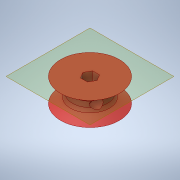
# Autodesk Inventor part: RoundShaftSpoolForArmV01
Saved by Autodesk Inventor 2022.2 (Build 262287010, 287A)
## iProperties
Created: 2019-02-24
Part Number: RoundShaftSpoolForArmV01
Material: PC/ABS Plastic
Document SubType Name: Modeling
Designer: steele
Density: 0.357273 g/cm^3
Appearance: Smooth - Red
holeForString: 0.200 in
stringDiameter: 0.120 in
clearanceForString: 0.080 in
clearanceForHexShaft: 0.020 in
spoolInteriorDiameter: 1.500 in
spoolInteriroRadius: 0.750 in
spoolExteriorDiameter: 2.500 in
spoolExteriorRadius: 1.250 in
hexHoleChamfer: 0.063 in
stringHoleCenterFromHexShaft: 0.360 in
textCircleDiameter: 1.875 in
textHeight: 0.180 in
textDepth: 0.050 in
Author: steele
Autodesk Inventor part; units mm, degrees
ref_plane "XZ Plane" through (0, 0, 0) normal (0, 1, 0) x (-1, 0, 0)
ref_plane "XY Plane" through (0, 0, 0) normal (0, 0, 1) x (1, 0, 0)
sketch "Sketch15" plane through (0, 0, 0) normal (0, 0, 1) x (1, 0, 0)
  line L0 (31.75, 0) -> (31.75, 50.8) construction
  line L1 (12.065, 0) -> (31.75, 0)
  line L2 (19.05, 0) -> (19.05, 50.8) construction
  line L3 (0, 50.8) -> (0, 0)
  line L4 (19.05, 12.7) -> (31.75, 12.7) construction
  line L5 (31.75, 0) -> (19.05, 7.3323)
  line L6 (31.75, 25.4) -> (19.05, 18.0677)
  line L7 (19.05, 18.0677) -> (31.75, 18.0677) construction
  line L8 (19.05, 18.0677) -> (19.05, 7.3323)
  line L9 (31.75, 25.4) -> (19.05, 32.7323)
  line L10 (19.05, 32.7323) -> (19.05, 43.4677)
  line L11 (19.05, 43.4677) -> (31.75, 50.8)
  line L12 (31.75, 25.4) -> (19.05, 25.4) construction
  line L13 (19.05, 43.4677) -> (31.75, 43.4677) construction
  line L14 (12.065, 0) -> (0, 0)
  line L15 (31.75, 50.8) -> (0, 50.8)
  dimension "d86" = 50.8
  dimension "d89" = 25.4
  dimension "centerLineForSpool" = 12.7
  dimension "d93" = 30
  dimension "d94" = 30
  dimension "d95" = 30
  dimension "d96" = 30
  dimension "d156" = 31.75
  dimension "d158" = 31.75
  constraints: 32 end point, 9 point on line, 3 horizontal, 2 midpoint, 2 perpendicular, 1 collinear, 1 vertical
  measures "d86" distance of L0.start L0.end
  measures "d89" distance from line of L6.start L1
  measures "centerLineForSpool" distance from line of L4.start L1
  measures "d93" angle of L5 L1
  measures "d94" angle of L6 L7
  measures "d95" angle of L9 L12
  measures "d96" angle of L11 L13
  measures "d156" distance from line of L0.end L3
  measures "d158" distance from line of L0.start L3
revolve "Revolution2" add sketch "Sketch15" angle 360 about axis through (0, 50.8, 0) along (0, -1, 0)
sketch "Sketch16" plane through (0, 0, 0) normal (0, -1, 0) x (1, 0, 0)
  line L0 (-7.6256, 0) -> (-3.8128, 6.604)
  line L1 (-3.8128, 6.604) -> (3.8128, 6.604)
  line L2 (3.8128, 6.604) -> (7.6256, 0)
  line L3 (7.6256, 0) -> (3.8128, -6.604)
  line L4 (3.8128, -6.604) -> (-3.8128, -6.604)
  line L5 (-3.8128, -6.604) -> (-7.6256, 0)
  point P0 (0, 0)
  point P1 (0, 0)
  dimension "d103" = 13.208
  constraints: 12 end point, 1 coincident, 1 horizontal, 13 other
  measures "d103" distance between parallel lines of L1 L4
extrude "Extrusion11" cut sketch "Sketch16" against normal through all
sketch "Sketch17" plane through (0, 0, 0) normal (1, 0, 0) x (0, 1, 0)
  circle A0 centre (38.1, 9.144) radius 2.54
  circle A1 centre (12.7, 9.144) radius 2.54
  line L0 (0, 31.75) -> (0, -31.75) projected
  line L1 (50.8, 31.75) -> (50.8, -31.75) projected
  line L2 (0, 6.604) -> (50.8, 6.604) projected
  point P0 (0, 0)
  point P1 (50.8, -31.75)
  point P2 (69.85, 6.858)
  point P3 (72.39, 6.858)
  point P4 (50.8, 6.604)
  dimension "d110" = 12.7
  dimension "d111" = 12.7
  dimension "d112" = 5.08
  constraints: 2 centre point, 1 equal radius, 4 other
  measures "d110" distance from line of A1.centre L0
  measures "d112" diameter of A0
extrude "Extrusion13" cut sketch "Sketch17" along normal through all both and the other way through all
ref_plane "Work Plane4" through (-19.05, 0, 0) normal (1, 0, 0) x (0, 1, 0)
sketch "Sketch22" plane through (-19.05, 0, 0) normal (1, 0, 0) x (0, 1, 0)
  spline S0 degree 8 poles (40.64, 9.144) (40.64, 9.42) (40.6057, 9.6896) (40.54, 9.9488) (40.4456, 10.1945) (40.3253, 10.4241) (40.1822, 10.6353) (40.019, 10.8263) (39.6643, 11.1594) (39.4723, 11.3044) (39.2651, 11.4282) (39.0456, 11.5293) (38.8165, 11.6061) (38.5806, 11.6579) (38.3408, 11.684) (37.8188, 11.684) (37.5395, 11.6484) (37.2666, 11.5781) (37.0042, 11.4743) (36.7566, 11.3384) (36.5278, 11.1726) (36.322, 10.9796) (35.9648, 10.5477) (35.8095, 10.305) (35.6834, 10.0377) (35.5915, 9.75) (35.5382, 9.4472) (35.5271, 9.1354) (35.5605, 8.8213) (35.7533, 8.0702) (35.9537, 7.6667) (36.2256, 7.316) (36.5542, 7.0287) (36.9234, 6.8124) (37.3159, 6.6712) (37.7136, 6.604) (38.3775, 6.604) (38.6564, 6.6386) (38.9325, 6.7085) (39.2015, 6.8141) (39.4588, 6.9552) (39.6993, 7.1318) (39.9175, 7.3429) (40.2331, 7.7498) (40.3461, 7.9265) (40.4431, 8.1154) (40.522, 8.3139) (40.5815, 8.5192) (40.6208, 8.7281) (40.64, 8.9374) (40.64, 9.144) knots 0 0 0 0 0 0 0 0 0 0.12897 0.12897 0.12897 0.12897 0.12897 0.12897 0.12897 0.253758 0.253758 0.253758 0.253758 0.253758 0.253758 0.253758 0.399502 0.399502 0.399502 0.399502 0.399502 0.399502 0.399502 0.544455 0.544455 0.544455 0.544455 0.544455 0.544455 0.544455 0.751871 0.751871 0.751871 0.751871 0.751871 0.751871 0.751871 0.90085 0.90085 0.90085 0.90085 0.90085 0.90085 0.90085 1 1 1 1 1 1 1 1 1 projected
  circle A0 centre (38.1, 9.144) radius 4.7625
  circle A1 centre (38.1, 9.144) radius 2.54 construction
  line L0 (38.1, 6.604) -> (12.7, 6.604) construction
  line L1 (50.8, 31.75) -> (50.8, -31.75) construction
  point P0 (0, 0)
  point P1 (69.85, 6.858)
  point P2 (50.8, -31.75)
  point P3 (72.39, 6.858)
  point P4 (12.7, 6.604)
  dimension "d121" = 12.7
  dimension "d122" = 5.08
  dimension "d125" = 9.525
  constraints: 2 centre point, 1 concentric, 1 vertical alignment, 3 other
  measures "d122" diameter of A1
  measures "d125" diameter of A0
extrude "Extrusion16" cut sketch "Sketch22" along normal blind 11.1125
ref_plane "Work Plane5" through (19.05, 0, 0) normal (1, 0, 0) x (0, 1, 0)
sketch "Sketch23" plane through (19.05, 0, 0) normal (1, 0, 0) x (0, 1, 0)
  line L0 (12.7, 6.604) -> (38.1, 6.604) projected
  circle A0 centre (12.7, 9.144) radius 2.54 construction
  line L1 (0, 31.75) -> (0, -31.75) projected
  circle A1 centre (12.7, 9.144) radius 4.7625
  point P0 (0, 0)
  dimension "d127" = 5.08
  dimension "d128" = 12.7
  dimension "d129" = 9.525
  constraints: 2 centre point, 1 coincident, 1 tangent
  measures "d127" diameter of A0
  measures "d128" distance from line of A0.centre L1
  measures "d129" diameter of A1
extrude "Extrusion17" cut sketch "Sketch23" against normal blind 11.1125
chamfer "Chamfer12" distance 2.3813 angle 45 4 edges at (-19.05, 43.4677, 0) (-19.05, 32.7323, 0) (-19.05, 18.0677, 0) (-19.05, 7.3323, 0)
ref_plane "Work Plane6" through (0, 25.4, 0) normal (0, -1, 0) x (1, 0, 0)
sketch "Sketch26" plane through (0, 0, 0) normal (0, -1, 0) x (1, 0, 0)
  circle A0 centre (0, 0) radius 23.8125 construction
  line L0 (-23.5941, 3.5966) -> (-23.6743, 2.6429)
  line L1 (-23.6743, 2.6429) -> (-25.3572, 2.7844)
  line L2 (-25.3572, 2.7844) -> (-25.4662, 1.4891)
  line L3 (-25.4662, 1.4891) -> (-23.7832, 1.3476)
  line L4 (-23.7832, 1.3476) -> (-23.8634, 0.3938)
  line L5 (-23.8634, 0.3938) -> (-27.66, 0.713)
  line L6 (-27.66, 0.713) -> (-27.5798, 1.6668)
  line L7 (-27.5798, 1.6668) -> (-26.1892, 1.5499)
  line L8 (-26.1892, 1.5499) -> (-26.0803, 2.8452)
  line L9 (-26.0803, 2.8452) -> (-27.4709, 2.9621)
  line L10 (-27.4709, 2.9621) -> (-27.3907, 3.9159)
  line L11 (-27.3907, 3.9159) -> (-23.5941, 3.5966)
  spline S0 degree 2 poles (-23.0339, 5.7334) (-23.2221, 4.9404) (-24.1795, 4.2759) (-24.8794, 4.442) knots 0 0 0 1 2 2 2
  spline S1 degree 2 poles (-24.8794, 4.442) (-25.5644, 4.6046) (-26.1947, 5.5856) (-26.0264, 6.2946) knots 0 0 0 1 2 2 2
  spline S2 degree 2 poles (-26.0264, 6.2946) (-25.8745, 6.9344) (-25.0266, 7.4186) (-24.3837, 7.266) knots 0 0 0 1 2 2 2
  line L12 (-24.3837, 7.266) -> (-24.0683, 7.1912)
  line L13 (-24.0683, 7.1912) -> (-24.5225, 5.2776)
  spline S3 degree 2 poles (-24.5225, 5.2776) (-24.3244, 5.2432) (-24.0325, 5.3231) (-23.9273, 5.4187) knots 0 0 0 1 2 2 2
  spline S4 degree 2 poles (-23.9273, 5.4187) (-23.8228, 5.5113) (-23.6854, 5.7961) (-23.6433, 5.9733) knots 0 0 0 1 2 2 2
  spline S5 degree 2 poles (-23.6433, 5.9733) (-23.6077, 6.1235) (-23.6039, 6.4336) (-23.6318, 6.5703) knots 0 0 0 1 2 2 2
  spline S6 degree 2 poles (-23.6318, 6.5703) (-23.6512, 6.6891) (-23.7195, 6.8958) (-23.748, 6.9628) knots 0 0 0 1 2 2 2
  line L14 (-23.748, 6.9628) -> (-23.7259, 7.056)
  line L15 (-23.7259, 7.056) -> (-23.005, 6.8848)
  spline S7 degree 2 poles (-23.005, 6.8848) (-22.9886, 6.7667) (-22.9578, 6.5754) (-22.9589, 6.4106) knots 0 0 0 1 2 2 2
  spline S8 degree 2 poles (-22.9589, 6.4106) (-22.9533, 6.2601) (-22.9825, 5.9497) (-23.0339, 5.7334) knots 0 0 0 1 2 2 2
  spline S9 degree 2 poles (-24.7979, 6.4568) (-25.0757, 6.5164) (-25.4249, 6.3422) (-25.484, 6.0928) knots 0 0 0 1 2 2 2
  spline S10 degree 2 poles (-25.484, 6.0928) (-25.5446, 5.8375) (-25.3067, 5.4764) (-25.0489, 5.3993) knots 0 0 0 1 2 2 2
  line L16 (-25.0489, 5.3993) -> (-24.7979, 6.4568)
  line L17 (-21.6776, 9.9814) -> (-22.0524, 9.0008)
  line L18 (-22.0524, 9.0008) -> (-23.0175, 8.7846)
  line L19 (-23.0175, 8.7846) -> (-22.4481, 7.9654)
  line L20 (-22.4481, 7.9654) -> (-22.8152, 7.005)
  line L21 (-22.8152, 7.005) -> (-23.781, 8.508)
  line L22 (-23.781, 8.508) -> (-25.4936, 8.0486)
  line L23 (-25.4936, 8.0486) -> (-25.1188, 9.0292)
  line L24 (-25.1188, 9.0292) -> (-24.1714, 9.2422)
  line L25 (-24.1714, 9.2422) -> (-24.7341, 10.0357)
  line L26 (-24.7341, 10.0357) -> (-24.367, 10.9961)
  line L27 (-24.367, 10.9961) -> (-23.4176, 9.5193)
  line L28 (-23.4176, 9.5193) -> (-21.6776, 9.9814)
  line L29 (-22.6697, 14.9203) -> (-22.7047, 14.8621)
  spline S11 degree 2 poles (-22.7047, 14.8621) (-22.745, 14.825) (-22.9002, 14.6625) (-22.9495, 14.5805) knots 0 0 0 1 2 2 2
  spline S12 degree 2 poles (-22.9495, 14.5805) (-23.0894, 14.3476) (-23.0218, 14.0764) (-22.7862, 13.9349) knots 0 0 0 1 2 2 2
  line L30 (-22.7862, 13.9349) -> (-22.7677, 13.9238)
  line L31 (-22.7677, 13.9238) -> (-22.4004, 14.5352)
  line L32 (-22.4004, 14.5352) -> (-21.8658, 14.214)
  line L33 (-21.8658, 14.214) -> (-22.2172, 13.6291)
  line L34 (-22.2172, 13.6291) -> (-20.2877, 12.4701)
  line L35 (-20.2877, 12.4701) -> (-20.7488, 11.7025)
  line L36 (-20.7488, 11.7025) -> (-22.6782, 12.8616)
  line L37 (-22.6782, 12.8616) -> (-22.8627, 12.5546)
  line L38 (-22.8627, 12.5546) -> (-23.3973, 12.8757)
  line L39 (-23.3973, 12.8757) -> (-23.2129, 13.1827)
  line L40 (-23.2129, 13.1827) -> (-23.2817, 13.2241)
  spline S13 degree 2 poles (-23.2817, 13.2241) (-23.7316, 13.4944) (-23.8969, 14.2384) (-23.6076, 14.7201) knots 0 0 0 1 2 2 2
  spline S14 degree 2 poles (-23.6076, 14.7201) (-23.5074, 14.8868) (-23.3103, 15.161) (-23.2255, 15.2542) knots 0 0 0 1 2 2 2
  line L41 (-23.2255, 15.2542) -> (-22.6697, 14.9203)
  spline S15 degree 2 poles (-19.1464, 16.5254) (-18.5825, 16.0937) (-18.4064, 14.9829) (-18.8361, 14.4215) knots 0 0 0 1 2 2 2
  spline S16 degree 2 poles (-18.8361, 14.4215) (-19.2641, 13.8625) (-20.3861, 13.7377) (-20.95, 14.1694) knots 0 0 0 1 2 2 2
  spline S17 degree 2 poles (-20.95, 14.1694) (-21.5188, 14.6048) (-21.6887, 15.7186) (-21.2608, 16.2776) knots 0 0 0 1 2 2 2
  spline S18 degree 2 poles (-21.2608, 16.2776) (-20.8329, 16.8366) (-19.7127, 16.9589) (-19.1464, 16.5254) knots 0 0 0 1 2 2 2
  spline S19 degree 2 poles (-19.6989, 15.7935) (-19.9024, 15.9493) (-20.2252, 16.0914) (-20.3511, 16.0945) knots 0 0 0 1 2 2 2
  spline S20 degree 2 poles (-20.3511, 16.0945) (-20.4857, 16.0964) (-20.6739, 15.9877) (-20.7509, 15.8872) knots 0 0 0 1 2 2 2
  spline S21 degree 2 poles (-20.7509, 15.8872) (-20.8259, 15.7892) (-20.8853, 15.5897) (-20.8508, 15.4621) knots 0 0 0 1 2 2 2
  spline S22 degree 2 poles (-20.8508, 15.4621) (-20.8192, 15.3408) (-20.5985, 15.0551) (-20.3877, 14.8937) knots 0 0 0 1 2 2 2
  spline S23 degree 2 poles (-20.3877, 14.8937) (-20.1793, 14.7342) (-19.8693, 14.6058) (-19.7477, 14.6021) knots 0 0 0 1 2 2 2
  spline S24 degree 2 poles (-19.7477, 14.6021) (-19.6261, 14.5985) (-19.4212, 14.7138) (-19.3423, 14.8167) knots 0 0 0 1 2 2 2
  spline S25 degree 2 poles (-19.3423, 14.8167) (-19.2766, 14.9025) (-19.2151, 15.1354) (-19.2473, 15.2456) knots 0 0 0 1 2 2 2
  spline S26 degree 2 poles (-19.2473, 15.2456) (-19.2862, 15.3726) (-19.4832, 15.6283) (-19.6989, 15.7935) knots 0 0 0 1 2 2 2
  line L42 (-17.7806, 18.7813) -> (-17.8322, 18.728)
  spline S27 degree 2 poles (-17.8322, 18.728) (-17.882, 18.7032) (-18.0305, 18.5763) (-18.1121, 18.4919) knots 0 0 0 1 2 2 2
  spline S28 degree 2 poles (-18.1121, 18.4919) (-18.2087, 18.3921) (-18.3656, 18.11) (-18.4266, 17.9671) knots 0 0 0 1 2 2 2
  line L43 (-18.4266, 17.9671) -> (-17.0441, 16.6297)
  line L44 (-17.0441, 16.6297) -> (-17.6666, 15.9861)
  line L45 (-17.6666, 15.9861) -> (-19.7326, 17.9847)
  line L46 (-19.7326, 17.9847) -> (-19.11, 18.6282)
  line L47 (-19.11, 18.6282) -> (-18.8127, 18.3406)
  spline S29 degree 2 poles (-18.8127, 18.3406) (-18.8097, 18.4236) (-18.7837, 18.6992) (-18.7592, 18.8) knots 0 0 0 1 2 2 2
  spline S30 degree 2 poles (-18.7592, 18.8) (-18.7326, 18.9118) (-18.6122, 19.1562) (-18.5328, 19.2383) knots 0 0 0 1 2 2 2
  spline S31 degree 2 poles (-18.5328, 19.2383) (-18.5027, 19.2693) (-18.4232, 19.3427) (-18.3909, 19.3716) knots 0 0 0 1 2 2 2
  line L48 (-18.3909, 19.3716) -> (-17.7806, 18.7813)
  line L49 (-15.2117, 18.4111) -> (-16.3547, 22.2669)
  line L50 (-16.3547, 22.2669) -> (-15.5018, 22.8682)
  line L51 (-15.5018, 22.8682) -> (-12.2542, 20.496)
  line L52 (-12.2542, 20.496) -> (-13.0592, 19.9285)
  line L53 (-13.0592, 19.9285) -> (-13.7018, 20.4275)
  line L54 (-13.7018, 20.4275) -> (-14.6809, 19.7372)
  line L55 (-14.6809, 19.7372) -> (-14.4295, 18.9626)
  line L56 (-14.4295, 18.9626) -> (-15.2117, 18.4111)
  line L57 (-14.2719, 20.8718) -> (-15.3157, 21.6772)
  line L58 (-15.3157, 21.6772) -> (-14.9103, 20.4217)
  line L59 (-14.9103, 20.4217) -> (-14.2719, 20.8718)
  line L60 (-11.17, 23.3264) -> (-11.2354, 23.2915)
  spline S32 degree 2 poles (-11.2354, 23.2915) (-11.2904, 23.2831) (-11.4707, 23.2078) (-11.5742, 23.1525) knots 0 0 0 1 2 2 2
  spline S33 degree 2 poles (-11.5742, 23.1525) (-11.6967, 23.0871) (-11.9325, 22.8666) (-12.0344, 22.7492) knots 0 0 0 1 2 2 2
  line L61 (-12.0344, 22.7492) -> (-11.1282, 21.0525)
  line L62 (-11.1282, 21.0525) -> (-11.918, 20.6307)
  line L63 (-11.918, 20.6307) -> (-13.2722, 23.1662)
  line L64 (-13.2722, 23.1662) -> (-12.4824, 23.5881)
  line L65 (-12.4824, 23.5881) -> (-12.2874, 23.2231)
  spline S34 degree 2 poles (-12.2874, 23.2231) (-12.2592, 23.3012) (-12.15, 23.5556) (-12.0957, 23.644) knots 0 0 0 1 2 2 2
  spline S35 degree 2 poles (-12.0957, 23.644) (-12.0362, 23.7423) (-11.8467, 23.938) (-11.7459, 23.9919) knots 0 0 0 1 2 2 2
  spline S36 degree 2 poles (-11.7459, 23.9919) (-11.7078, 24.0122) (-11.6096, 24.0577) (-11.57, 24.0753) knots 0 0 0 1 2 2 2
  line L66 (-11.57, 24.0753) -> (-11.17, 23.3264)
  line L67 (-6.7012, 22.8857) -> (-7.1777, 24.24)
  spline S37 degree 2 poles (-7.1777, 24.24) (-7.2484, 24.441) (-7.3593, 24.7096) (-7.425, 24.7847) knots 0 0 0 1 2 2 2
  spline S38 degree 2 poles (-7.425, 24.7847) (-7.4936, 24.8587) (-7.6727, 24.8841) (-7.8096, 24.8359) knots 0 0 0 1 2 2 2
  spline S39 degree 2 poles (-7.8096, 24.8359) (-7.9057, 24.8021) (-8.0624, 24.6521) (-8.1454, 24.5345) knots 0 0 0 1 2 2 2
  line L68 (-8.1454, 24.5345) -> (-7.4701, 22.6152)
  line L69 (-7.4701, 22.6152) -> (-8.3205, 22.3159)
  line L70 (-8.3205, 22.3159) -> (-8.797, 23.6702)
  spline S40 degree 2 poles (-8.797, 23.6702) (-8.8667, 23.8682) (-8.9816, 24.1388) (-9.0473, 24.2139) knots 0 0 0 1 2 2 2
  spline S41 degree 2 poles (-9.0473, 24.2139) (-9.1159, 24.2879) (-9.295, 24.3133) (-9.4319, 24.2651) knots 0 0 0 1 2 2 2
  spline S42 degree 2 poles (-9.4319, 24.2651) (-9.5338, 24.2292) (-9.701, 24.0624) (-9.7706, 23.9626) knots 0 0 0 1 2 2 2
  line L71 (-9.7706, 23.9626) -> (-9.0952, 22.0433)
  line L72 (-9.0952, 22.0433) -> (-9.9398, 21.7461)
  line L73 (-9.9398, 21.7461) -> (-10.894, 24.4576)
  line L74 (-10.894, 24.4576) -> (-10.0493, 24.7548)
  line L75 (-10.0493, 24.7548) -> (-9.9438, 24.4548)
  spline S43 degree 2 poles (-9.9438, 24.4548) (-9.7985, 24.7023) (-9.4983, 25.0305) (-9.2682, 25.1115) knots 0 0 0 1 2 2 2
  spline S44 degree 2 poles (-9.2682, 25.1115) (-9.0206, 25.1986) (-8.559, 25.0959) (-8.377, 24.8949) knots 0 0 0 1 2 2 2
  spline S45 degree 2 poles (-8.377, 24.8949) (-8.2152, 25.2071) (-7.8702, 25.6034) (-7.6489, 25.6813) knots 0 0 0 1 2 2 2
  spline S46 degree 2 poles (-7.6489, 25.6813) (-7.4596, 25.7479) (-7.1176, 25.7341) (-6.9726, 25.6476) knots 0 0 0 1 2 2 2
  spline S47 degree 2 poles (-6.9726, 25.6476) (-6.8129, 25.5565) (-6.5732, 25.2383) (-6.4718, 24.9499) knots 0 0 0 1 2 2 2
  line L76 (-6.4718, 24.9499) -> (-5.8507, 23.185)
  line L77 (-5.8507, 23.185) -> (-6.7012, 22.8857)
  line L78 (-4.5034, 25.2866) -> (-5.3911, 25.1122)
  line L79 (-5.3911, 25.1122) -> (-5.5851, 26.0999)
  line L80 (-5.5851, 26.0999) -> (-4.6974, 26.2742)
  line L81 (-4.6974, 26.2742) -> (-4.5034, 25.2866)
  line L82 (-4.1435, 23.4536) -> (-5.0311, 23.2793)
  line L83 (-5.0311, 23.2793) -> (-5.2251, 24.267)
  line L84 (-5.2251, 24.267) -> (-4.3374, 24.4413)
  line L85 (-4.3374, 24.4413) -> (-4.1435, 23.4536)
  spline S48 degree 2 poles (0.9633, 25.7414) (0.973, 25.2474) (0.8301, 24.5035) (0.659, 24.25) knots 0 0 0 1 2 2 2
  spline S49 degree 2 poles (0.659, 24.25) (0.491, 23.9997) (-0.0628, 23.7356) (-0.4641, 23.7277) knots 0 0 0 1 2 2 2
  spline S50 degree 2 poles (-0.4641, 23.7277) (-0.8684, 23.7198) (-1.4291, 23.962) (-1.61, 24.2117) knots 0 0 0 1 2 2 2
  spline S51 degree 2 poles (-1.61, 24.2117) (-1.7908, 24.4582) (-1.9627, 25.1898) (-1.9724, 25.6837) knots 0 0 0 1 2 2 2
  spline S52 degree 2 poles (-1.9724, 25.6837) (-1.9823, 26.19) (-1.8389, 26.9093) (-1.665, 27.1721) knots 0 0 0 1 2 2 2
  spline S53 degree 2 poles (-1.665, 27.1721) (-1.4909, 27.4287) (-0.9309, 27.6868) (-0.5419, 27.6944) knots 0 0 0 1 2 2 2
  spline S54 degree 2 poles (-0.5419, 27.6944) (-0.1313, 27.7024) (0.4232, 27.4539) (0.6042, 27.2012) knots 0 0 0 1 2 2 2
  spline S55 degree 2 poles (0.6042, 27.2012) (0.782, 26.9545) (0.9539, 26.2198) (0.9633, 25.7414) knots 0 0 0 1 2 2 2
  spline S56 degree 2 poles (0.0032, 25.7225) (-0.0106, 26.4294) (-0.2534, 26.996) (-0.5281, 26.9906) knots 0 0 0 1 2 2 2
  spline S57 degree 2 poles (-0.5281, 26.9906) (-0.8028, 26.9852) (-1.0262, 26.4095) (-1.0123, 25.6995) knots 0 0 0 1 2 2 2
  spline S58 degree 2 poles (-1.0123, 25.6995) (-0.9986, 25.0019) (-0.7526, 24.4261) (-0.4779, 24.4315) knots 0 0 0 1 2 2 2
  spline S59 degree 2 poles (-0.4779, 24.4315) (-0.2062, 24.4368) (0.017, 25.0218) (0.0032, 25.7225) knots 0 0 0 1 2 2 2
  line L86 (2.4635, 23.689) -> (1.5621, 23.7655)
  line L87 (1.5621, 23.7655) -> (1.6472, 24.7685)
  line L88 (1.6472, 24.7685) -> (2.5486, 24.6919)
  line L89 (2.5486, 24.6919) -> (2.4635, 23.689)
  spline S60 degree 2 poles (6.122, 24.3872) (6.0657, 24.093) (5.7705, 23.634) (5.5391, 23.4927) knots 0 0 0 1 2 2 2
  spline S61 degree 2 poles (5.5391, 23.4927) (5.3078, 23.3515) (4.7303, 23.2577) (4.336, 23.3331) knots 0 0 0 1 2 2 2
  spline S62 degree 2 poles (4.336, 23.3331) (3.9181, 23.4162) (3.3438, 23.6675) (3.1635, 23.7931) knots 0 0 0 1 2 2 2
  line L90 (3.1635, 23.7931) -> (3.3195, 24.6089)
  line L91 (3.3195, 24.6089) -> (3.4045, 24.5927)
  spline S63 degree 2 poles (3.4045, 24.5927) (3.4697, 24.5393) (3.6259, 24.4026) (3.758, 24.3207) knots 0 0 0 1 2 2 2
  spline S64 degree 2 poles (3.758, 24.3207) (3.8815, 24.2436) (4.1441, 24.1211) (4.3109, 24.0892) knots 0 0 0 1 2 2 2
  spline S65 degree 2 poles (4.3109, 24.0892) (4.4565, 24.0613) (4.8101, 24.0692) (4.9317, 24.1465) knots 0 0 0 1 2 2 2
  spline S66 degree 2 poles (4.9317, 24.1465) (5.022, 24.2078) (5.1423, 24.3765) (5.1719, 24.5312) knots 0 0 0 1 2 2 2
  spline S67 degree 2 poles (5.1719, 24.5312) (5.1974, 24.6646) (5.1242, 24.8735) (5.0473, 24.948) knots 0 0 0 1 2 2 2
  spline S68 degree 2 poles (5.0473, 24.948) (4.9362, 25.0572) (4.5816, 25.1754) (4.4512, 25.2003) knots 0 0 0 1 2 2 2
  spline S69 degree 2 poles (4.4512, 25.2003) (4.245, 25.2398) (3.841, 25.2479) (3.6915, 25.2387) knots 0 0 0 1 2 2 2
  line L92 (3.6915, 25.2387) -> (3.6096, 25.2544)
  line L93 (3.6096, 25.2544) -> (4.0116, 27.356)
  line L94 (4.0116, 27.356) -> (6.4923, 26.8814)
  line L95 (6.4923, 26.8814) -> (6.3571, 26.1749)
  line L96 (6.3571, 26.1749) -> (4.765, 26.4794)
  line L97 (4.765, 26.4794) -> (4.6461, 25.8577)
  spline S70 degree 2 poles (4.6461, 25.8577) (4.7231, 25.8493) (4.9335, 25.8153) (4.9911, 25.8043) knots 0 0 0 1 2 2 2
  spline S71 degree 2 poles (4.9911, 25.8043) (5.261, 25.7527) (5.695, 25.5565) (5.8524, 25.4101) knots 0 0 0 1 2 2 2
  spline S72 degree 2 poles (5.8524, 25.4101) (6.038, 25.23) (6.1858, 24.7207) (6.122, 24.3872) knots 0 0 0 1 2 2 2
  line L98 (9.1285, 22.0456) -> (6.4783, 22.9502)
  line L99 (6.4783, 22.9502) -> (6.6788, 23.5375)
  spline S73 degree 2 poles (6.6788, 23.5375) (7.1065, 23.6917) (7.8058, 23.9815) (8.0802, 24.126) knots 0 0 0 1 2 2 2
  spline S74 degree 2 poles (8.0802, 24.126) (8.4408, 24.3128) (8.8221, 24.6557) (8.8979, 24.8778) knots 0 0 0 1 2 2 2
  spline S75 degree 2 poles (8.8979, 24.8778) (8.9837, 25.1291) (8.7745, 25.5006) (8.5057, 25.5924) knots 0 0 0 1 2 2 2
  spline S76 degree 2 poles (8.5057, 25.5924) (8.3684, 25.6393) (8.1, 25.6558) (7.9564, 25.6461) knots 0 0 0 1 2 2 2
  spline S77 degree 2 poles (7.9564, 25.6461) (7.8147, 25.6325) (7.5995, 25.5755) (7.5457, 25.5612) knots 0 0 0 1 2 2 2
  line L100 (7.5457, 25.5612) -> (7.4756, 25.5852)
  line L101 (7.4756, 25.5852) -> (7.7439, 26.3712)
  spline S78 degree 2 poles (7.7439, 26.3712) (7.9207, 26.3924) (8.6213, 26.3229) (8.9222, 26.2201) knots 0 0 0 1 2 2 2
  spline S79 degree 2 poles (8.9222, 26.2201) (9.5651, 26.0007) (10.03, 25.2026) (9.8534, 24.6854) knots 0 0 0 1 2 2 2
  spline S80 degree 2 poles (9.8534, 24.6854) (9.7447, 24.3669) (9.2343, 23.856) (8.7669, 23.6241) knots 0 0 0 1 2 2 2
  spline S81 degree 2 poles (8.7669, 23.6241) (8.4739, 23.4827) (7.9472, 23.2873) (7.8327, 23.248) knots 0 0 0 1 2 2 2
  line L102 (7.8327, 23.248) -> (9.3609, 22.7264)
  line L103 (9.3609, 22.7264) -> (9.1285, 22.0456)
  spline S82 degree 2 poles (12.9309, 22.2786) (12.7077, 21.8379) (12.2324, 21.248) (11.9624, 21.1045) knots 0 0 0 1 2 2 2
  spline S83 degree 2 poles (11.9624, 21.1045) (11.6965, 20.9623) (11.0836, 20.9889) (10.7255, 21.1703) knots 0 0 0 1 2 2 2
  spline S84 degree 2 poles (10.7255, 21.1703) (10.3647, 21.3531) (9.9833, 21.8301) (9.9407, 22.1354) knots 0 0 0 1 2 2 2
  spline S85 degree 2 poles (9.9407, 22.1354) (9.8967, 22.4381) (10.0883, 23.1648) (10.3116, 23.6054) knots 0 0 0 1 2 2 2
  spline S86 degree 2 poles (10.3116, 23.6054) (10.5404, 24.0571) (11.0045, 24.625) (11.2815, 24.7754) knots 0 0 0 1 2 2 2
  spline S87 degree 2 poles (11.2815, 24.7754) (11.5556, 24.9204) (12.1713, 24.8854) (12.5183, 24.7096) knots 0 0 0 1 2 2 2
  spline S88 degree 2 poles (12.5183, 24.7096) (12.8846, 24.524) (13.2577, 24.0443) (13.2989, 23.7362) knots 0 0 0 1 2 2 2
  spline S89 degree 2 poles (13.2989, 23.7362) (13.3401, 23.435) (13.1472, 22.7055) (12.9309, 22.2786) knots 0 0 0 1 2 2 2
  spline S90 degree 2 poles (12.0743, 22.7125) (12.3938, 23.3433) (12.4454, 23.9574) (12.2002, 24.0816) knots 0 0 0 1 2 2 2
  spline S91 degree 2 poles (12.2002, 24.0816) (11.9551, 24.2058) (11.4876, 23.8023) (11.1668, 23.1688) knots 0 0 0 1 2 2 2
  spline S92 degree 2 poles (11.1668, 23.1688) (10.8514, 22.5463) (10.7985, 21.9225) (11.0436, 21.7983) knots 0 0 0 1 2 2 2
  spline S93 degree 2 poles (11.0436, 21.7983) (11.286, 21.6755) (11.7576, 22.0873) (12.0743, 22.7125) knots 0 0 0 1 2 2 2
  line L104 (15.3435, 18.2391) -> (13.7194, 19.4901)
  line L105 (13.7194, 19.4901) -> (14.1244, 20.016)
  line L106 (14.1244, 20.016) -> (14.5574, 19.6825)
  line L107 (14.5574, 19.6825) -> (16.0722, 21.6491)
  line L108 (16.0722, 21.6491) -> (15.6393, 21.9826)
  line L109 (15.6393, 21.9826) -> (16.0444, 22.5085)
  line L110 (16.0444, 22.5085) -> (17.6685, 21.2574)
  line L111 (17.6685, 21.2574) -> (17.2634, 20.7315)
  line L112 (17.2634, 20.7315) -> (16.8305, 21.065)
  line L113 (16.8305, 21.065) -> (15.3156, 19.0984)
  line L114 (15.3156, 19.0984) -> (15.7486, 18.7649)
  line L115 (15.7486, 18.7649) -> (15.3435, 18.2391)
  spline S94 degree 2 poles (19.5844, 16.7619) (19.204, 16.387) (18.2786, 16.1294) (17.8688, 16.2241) knots 0 0 0 1 2 2 2
  spline S95 degree 2 poles (17.8688, 16.2241) (17.5244, 16.3008) (16.9554, 16.7197) (16.6802, 16.999) knots 0 0 0 1 2 2 2
  line L116 (16.6802, 16.999) -> (15.8435, 17.8477)
  line L117 (15.8435, 17.8477) -> (18.5569, 20.5223)
  line L118 (18.5569, 20.5223) -> (19.3849, 19.6824)
  spline S96 degree 2 poles (19.3849, 19.6824) (19.6667, 19.3965) (20.0861, 18.8259) (20.1621, 18.4673) knots 0 0 0 1 2 2 2
  spline S97 degree 2 poles (20.1621, 18.4673) (20.2529, 18.0321) (19.978, 17.1499) (19.5844, 16.7619) knots 0 0 0 1 2 2 2
  spline S98 degree 2 poles (18.8995, 17.4655) (19.1678, 17.7299) (19.3683, 18.2918) (19.2897, 18.5871) knots 0 0 0 1 2 2 2
  spline S99 degree 2 poles (19.2897, 18.5871) (19.2279, 18.7993) (18.9442, 19.1179) (18.7361, 19.329) knots 0 0 0 1 2 2 2
  line L119 (18.7361, 19.329) -> (18.7231, 19.3422)
  line L120 (18.7231, 19.3422) -> (17.0234, 17.6668)
  line L121 (17.0234, 17.6668) -> (17.0364, 17.6536)
  spline S100 degree 2 poles (17.0364, 17.6536) (17.2618, 17.4249) (17.5871, 17.1256) (17.8182, 17.0716) knots 0 0 0 1 2 2 2
  spline S101 degree 2 poles (17.8182, 17.0716) (18.0884, 17.0085) (18.6313, 17.2011) (18.8995, 17.4655) knots 0 0 0 1 2 2 2
  line L122 (19.1585, 14.149) -> (18.6073, 14.8664)
  line L123 (18.6073, 14.8664) -> (19.4054, 15.4796)
  line L124 (19.4054, 15.4796) -> (19.9566, 14.7623)
  line L125 (19.9566, 14.7623) -> (19.1585, 14.149)
  line L126 (20.6396, 15.2872) -> (20.0884, 16.0045)
  line L127 (20.0884, 16.0045) -> (20.8865, 16.6178)
  line L128 (20.8865, 16.6178) -> (21.4377, 15.9004)
  line L129 (21.4377, 15.9004) -> (20.6396, 15.2872)
  line L130 (21.7353, 9.8198) -> (20.5714, 12.0507)
  line L131 (20.5714, 12.0507) -> (21.1599, 12.3578)
  line L132 (21.1599, 12.3578) -> (21.5312, 11.646)
  line L133 (21.5312, 11.646) -> (23.3187, 12.5786)
  line L134 (23.3187, 12.5786) -> (22.9474, 13.2903)
  line L135 (22.9474, 13.2903) -> (23.4976, 13.5774)
  spline S102 degree 2 poles (23.4976, 13.5774) (23.579, 13.4214) (23.7815, 13.1335) (23.8738, 13.0633) knots 0 0 0 1 2 2 2
  spline S103 degree 2 poles (23.8738, 13.0633) (23.9843, 12.9851) (24.2305, 12.9603) (24.3731, 13.0208) knots 0 0 0 1 2 2 2
  line L136 (24.3731, 13.0208) -> (24.7587, 12.2817)
  line L137 (24.7587, 12.2817) -> (21.9611, 10.8221)
  line L138 (21.9611, 10.8221) -> (22.3238, 10.1268)
  line L139 (22.3238, 10.1268) -> (21.7353, 9.8198)
  line L140 (22.3098, 8.3373) -> (21.9772, 9.1786)
  line L141 (21.9772, 9.1786) -> (22.9132, 9.5487)
  line L142 (22.9132, 9.5487) -> (23.2458, 8.7074)
  line L143 (23.2458, 8.7074) -> (22.3098, 8.3373)
  spline S104 degree 2 poles (24.5633, 5.3718) (24.2748, 5.2913) (23.7323, 5.3514) (23.5029, 5.4957) knots 0 0 0 1 2 2 2
  spline S105 degree 2 poles (23.5029, 5.4957) (23.2735, 5.6401) (22.9324, 6.1154) (22.8245, 6.502) knots 0 0 0 1 2 2 2
  spline S106 degree 2 poles (22.8245, 6.502) (22.7129, 6.9132) (22.6823, 7.5394) (22.7146, 7.7568) knots 0 0 0 1 2 2 2
  line L144 (22.7146, 7.7568) -> (23.5146, 7.9801)
  line L145 (23.5146, 7.9801) -> (23.5378, 7.8969)
  spline S107 degree 2 poles (23.5378, 7.8969) (23.5191, 7.8147) (23.4661, 7.614) (23.4516, 7.4593) knots 0 0 0 1 2 2 2
  spline S108 degree 2 poles (23.4516, 7.4593) (23.4376, 7.3143) (23.4447, 7.0246) (23.4904, 6.861) knots 0 0 0 1 2 2 2
  spline S109 degree 2 poles (23.4904, 6.861) (23.5303, 6.7183) (23.6946, 6.4052) (23.818, 6.3306) knots 0 0 0 1 2 2 2
  spline S110 degree 2 poles (23.818, 6.3306) (23.9131, 6.277) (24.1178, 6.2444) (24.2694, 6.2867) knots 0 0 0 1 2 2 2
  spline S111 degree 2 poles (24.2694, 6.2867) (24.4003, 6.3233) (24.5548, 6.4818) (24.5872, 6.5838) knots 0 0 0 1 2 2 2
  spline S112 degree 2 poles (24.5872, 6.5838) (24.6356, 6.732) (24.5835, 7.1021) (24.5478, 7.23) knots 0 0 0 1 2 2 2
  spline S113 degree 2 poles (24.5478, 7.23) (24.4914, 7.4322) (24.3188, 7.7975) (24.2441, 7.9274) knots 0 0 0 1 2 2 2
  line L146 (24.2441, 7.9274) -> (24.2217, 8.0076)
  line L147 (24.2217, 8.0076) -> (26.2826, 8.583)
  line L148 (26.2826, 8.583) -> (26.9617, 6.1504)
  line L149 (26.9617, 6.1504) -> (26.2688, 5.957)
  line L150 (26.2688, 5.957) -> (25.8329, 7.5182)
  line L151 (25.8329, 7.5182) -> (25.2233, 7.348)
  spline S114 degree 2 poles (25.2233, 7.348) (25.25, 7.2753) (25.3132, 7.0718) (25.329, 7.0153) knots 0 0 0 1 2 2 2
  spline S115 degree 2 poles (25.329, 7.0153) (25.4029, 6.7506) (25.4204, 6.2747) (25.3593, 6.0685) knots 0 0 0 1 2 2 2
  spline S116 degree 2 poles (25.3593, 6.0685) (25.2807, 5.8222) (24.8904, 5.4632) (24.5633, 5.3718) knots 0 0 0 1 2 2 2
  line L152 (27.468, 4.2349) -> (25.9551, 4.1646)
  line L153 (25.9551, 4.1646) -> (25.8774, 4.6837)
  line L154 (25.8774, 4.6837) -> (27.3447, 5.0593)
  line L155 (27.3447, 5.0593) -> (27.468, 4.2349)
  line L156 (27.6275, 3.1692) -> (26.1145, 3.0989)
  line L157 (26.1145, 3.0989) -> (26.0369, 3.618)
  line L158 (26.0369, 3.618) -> (27.5041, 3.9937)
  line L159 (27.5041, 3.9937) -> (27.6275, 3.1692)
  spline S117 degree 2 poles (25.5799, -3.2348) (24.655, -3.1846) (23.651, -2.1407) (23.6975, -1.2836) knots 0 0 0 1 2 2 2
  spline S118 degree 2 poles (23.6975, -1.2836) (23.7441, -0.4235) (24.8671, 0.4989) (25.7797, 0.4494) knots 0 0 0 1 2 2 2
  spline S119 degree 2 poles (25.7797, 0.4494) (26.6953, 0.3998) (27.7089, -0.6385) (27.6622, -1.4986) knots 0 0 0 1 2 2 2
  spline S120 degree 2 poles (27.6622, -1.4986) (27.6157, -2.3557) (26.5017, -3.2848) (25.5799, -3.2348) knots 0 0 0 1 2 2 2
  spline S121 degree 2 poles (25.6334, -2.2482) (25.9756, -2.2668) (26.461, -2.1539) (26.6186, -2.0419) knots 0 0 0 1 2 2 2
  spline S122 degree 2 poles (26.6186, -2.0419) (26.7823, -1.9302) (26.9347, -1.6293) (26.9437, -1.4628) knots 0 0 0 1 2 2 2
  spline S123 degree 2 poles (26.9437, -1.4628) (26.9532, -1.287) (26.8424, -0.9935) (26.6893, -0.8522) knots 0 0 0 1 2 2 2
  spline S124 degree 2 poles (26.6893, -0.8522) (26.5476, -0.727) (26.0653, -0.5555) (25.7262, -0.5371) knots 0 0 0 1 2 2 2
  spline S125 degree 2 poles (25.7262, -0.5371) (25.3747, -0.5181) (24.9047, -0.6317) (24.741, -0.7435) knots 0 0 0 1 2 2 2
  spline S126 degree 2 poles (24.741, -0.7435) (24.5772, -0.8552) (24.4247, -1.1592) (24.4157, -1.3257) knots 0 0 0 1 2 2 2
  spline S127 degree 2 poles (24.4157, -1.3257) (24.4065, -1.4952) (24.5343, -1.8176) (24.6823, -1.94) knots 0 0 0 1 2 2 2
  spline S128 degree 2 poles (24.6823, -1.94) (24.8421, -2.0723) (25.2757, -2.2288) (25.6334, -2.2482) knots 0 0 0 1 2 2 2
  spline S129 degree 2 poles (24.6859, -7.4239) (24.1649, -7.3064) (23.4482, -6.6668) (23.3065, -6.2709) knots 0 0 0 1 2 2 2
  spline S130 degree 2 poles (23.3065, -6.2709) (23.185, -5.9396) (23.2301, -5.2345) (23.3163, -4.852) knots 0 0 0 1 2 2 2
  line L160 (23.3163, -4.852) -> (23.5785, -3.6894)
  line L161 (23.5785, -3.6894) -> (27.2952, -4.5276)
  line L162 (27.2952, -4.5276) -> (27.0357, -5.6781)
  spline S131 degree 2 poles (27.0357, -5.6781) (26.9474, -6.0697) (26.6938, -6.731) (26.4331, -6.9887) knots 0 0 0 1 2 2 2
  spline S132 degree 2 poles (26.4331, -6.9887) (26.116, -7.3001) (25.2251, -7.5455) (24.6859, -7.4239) knots 0 0 0 1 2 2 2
  spline S133 degree 2 poles (24.908, -6.4675) (25.2754, -6.5503) (25.8566, -6.4155) (26.0626, -6.1898) knots 0 0 0 1 2 2 2
  spline S134 degree 2 poles (26.0626, -6.1898) (26.2078, -6.0232) (26.3226, -5.6123) (26.3878, -5.3231) knots 0 0 0 1 2 2 2
  line L163 (26.3878, -5.3231) -> (26.3919, -5.3051)
  line L164 (26.3919, -5.3051) -> (24.0637, -4.78)
  line L165 (24.0637, -4.78) -> (24.0596, -4.798)
  spline S135 degree 2 poles (24.0596, -4.798) (23.989, -5.1113) (23.9129, -5.5467) (23.9923, -5.7704) knots 0 0 0 1 2 2 2
  spline S136 degree 2 poles (23.9923, -5.7704) (24.0852, -6.0319) (24.5405, -6.3846) (24.908, -6.4675) knots 0 0 0 1 2 2 2
  line L166 (22.2571, -8.4772) -> (22.5629, -7.6258)
  line L167 (22.5629, -7.6258) -> (23.5102, -7.966)
  line L168 (23.5102, -7.966) -> (23.2044, -8.8174)
  line L169 (23.2044, -8.8174) -> (22.2571, -8.4772)
  line L170 (24.0151, -9.1086) -> (24.3209, -8.2572)
  line L171 (24.3209, -8.2572) -> (25.2682, -8.5975)
  line L172 (25.2682, -8.5975) -> (24.9624, -9.4489)
  line L173 (24.9624, -9.4489) -> (24.0151, -9.1086)
  line L174 (20.0063, -12.9846) -> (21.2548, -10.7998)
  line L175 (21.2548, -10.7998) -> (21.8311, -11.1291)
  line L176 (21.8311, -11.1291) -> (21.4328, -11.8261)
  line L177 (21.4328, -11.8261) -> (23.1834, -12.8264)
  line L178 (23.1834, -12.8264) -> (23.5816, -12.1294)
  line L179 (23.5816, -12.1294) -> (24.1205, -12.4373)
  spline S137 degree 2 poles (24.1205, -12.4373) (24.0331, -12.5901) (23.9003, -12.916) (23.8911, -13.0317) knots 0 0 0 1 2 2 2
  spline S138 degree 2 poles (23.8911, -13.0317) (23.8849, -13.1669) (23.9971, -13.3875) (24.125, -13.4748) knots 0 0 0 1 2 2 2
  line L180 (24.125, -13.4748) -> (23.7114, -14.1986)
  line L181 (23.7114, -14.1986) -> (20.9718, -12.633)
  line L182 (20.9718, -12.633) -> (20.5827, -13.3139)
  line L183 (20.5827, -13.3139) -> (20.0063, -12.9846)
  line L184 (19.0692, -14.2689) -> (19.5974, -13.5345)
  line L185 (19.5974, -13.5345) -> (20.4146, -14.1222)
  line L186 (20.4146, -14.1222) -> (19.8864, -14.8566)
  line L187 (19.8864, -14.8566) -> (19.0692, -14.2689)
  spline S139 degree 2 poles (18.2255, -18.2038) (17.8566, -17.8752) (17.4081, -17.2647) (17.3384, -16.9669) knots 0 0 0 1 2 2 2
  spline S140 degree 2 poles (17.3384, -16.9669) (17.269, -16.6735) (17.4517, -16.0878) (17.7187, -15.7881) knots 0 0 0 1 2 2 2
  spline S141 degree 2 poles (17.7187, -15.7881) (17.9878, -15.4861) (18.5465, -15.2396) (18.8526, -15.2766) knots 0 0 0 1 2 2 2
  spline S142 degree 2 poles (18.8526, -15.2766) (19.1564, -15.3116) (19.8098, -15.6828) (20.1787, -16.0114) knots 0 0 0 1 2 2 2
  spline S143 degree 2 poles (20.1787, -16.0114) (20.5568, -16.3483) (20.9868, -16.9423) (21.0614, -17.2485) knots 0 0 0 1 2 2 2
  spline S144 degree 2 poles (21.0614, -17.2485) (21.1313, -17.5507) (20.9399, -18.1369) (20.6811, -18.4273) knots 0 0 0 1 2 2 2
  spline S145 degree 2 poles (20.6811, -18.4273) (20.4079, -18.7339) (19.8487, -18.9717) (19.5403, -18.9327) knots 0 0 0 1 2 2 2
  spline S146 degree 2 poles (19.5403, -18.9327) (19.2385, -18.8954) (18.5828, -18.5221) (18.2255, -18.2038) knots 0 0 0 1 2 2 2
  spline S147 degree 2 poles (18.8642, -17.4868) (19.3921, -17.9572) (19.9727, -18.1642) (20.1555, -17.959) knots 0 0 0 1 2 2 2
  spline S148 degree 2 poles (20.1555, -17.959) (20.3382, -17.7539) (20.0679, -17.1987) (19.5376, -16.7263) knots 0 0 0 1 2 2 2
  spline S149 degree 2 poles (19.5376, -16.7263) (19.0166, -16.2621) (18.4271, -16.0512) (18.2444, -16.2564) knots 0 0 0 1 2 2 2
  spline S150 degree 2 poles (18.2444, -16.2564) (18.0636, -16.4593) (18.3409, -17.0206) (18.8642, -17.4868) knots 0 0 0 1 2 2 2
  line L188 (18.404, -20.826) -> (17.5274, -19.5908)
  line L189 (17.5274, -19.5908) -> (17.9223, -19.245)
  line L190 (17.9223, -19.245) -> (19.0311, -20.2767)
  line L191 (19.0311, -20.2767) -> (18.404, -20.826)
  line L192 (17.5934, -21.5359) -> (16.7168, -20.3007)
  line L193 (16.7168, -20.3007) -> (17.1117, -19.9549)
  line L194 (17.1117, -19.9549) -> (18.2205, -20.9867)
  line L195 (18.2205, -20.9867) -> (17.5934, -21.5359)
  line L196 (10.3779, -21.4923) -> (11.2098, -21.019)
  line L197 (11.2098, -21.019) -> (12.0449, -22.4869)
  line L198 (12.0449, -22.4869) -> (13.1747, -21.8442)
  line L199 (13.1747, -21.8442) -> (12.3396, -20.3762)
  line L200 (12.3396, -20.3762) -> (13.1716, -19.903)
  line L201 (13.1716, -19.903) -> (15.0555, -23.2146)
  line L202 (15.0555, -23.2146) -> (14.2236, -23.6879)
  line L203 (14.2236, -23.6879) -> (13.5335, -22.4748)
  line L204 (13.5335, -22.4748) -> (12.4037, -23.1176)
  line L205 (12.4037, -23.1176) -> (13.0938, -24.3306)
  line L206 (13.0938, -24.3306) -> (12.2618, -24.8039)
  line L207 (12.2618, -24.8039) -> (10.3779, -21.4923)
  spline S151 degree 2 poles (8.6536, -22.1276) (9.1596, -21.921) (9.7931, -22.1493) (9.9868, -22.6237) knots 0 0 0 1 2 2 2
  line L208 (9.9868, -22.6237) -> (10.4945, -23.8672)
  line L209 (10.4945, -23.8672) -> (10.8118, -23.7376)
  line L210 (10.8118, -23.7376) -> (11.0476, -24.315)
  line L211 (11.0476, -24.315) -> (10.7303, -24.4445)
  line L212 (10.7303, -24.4445) -> (11.0408, -25.2049)
  line L213 (11.0408, -25.2049) -> (10.2118, -25.5434)
  line L214 (10.2118, -25.5434) -> (9.9014, -24.783)
  line L215 (9.9014, -24.783) -> (9.101, -25.1098)
  line L216 (9.101, -25.1098) -> (8.8652, -24.5324)
  line L217 (8.8652, -24.5324) -> (9.6656, -24.2056)
  line L218 (9.6656, -24.2056) -> (9.2793, -23.2595)
  spline S152 degree 2 poles (9.2793, -23.2595) (9.2221, -23.1194) (9.1311, -22.9131) (9.063, -22.8442) knots 0 0 0 1 2 2 2
  spline S153 degree 2 poles (9.063, -22.8442) (8.9948, -22.7753) (8.7865, -22.747) (8.6264, -22.8124) knots 0 0 0 1 2 2 2
  spline S154 degree 2 poles (8.6264, -22.8124) (8.5578, -22.8404) (8.3668, -22.9851) (8.3333, -23.0255) knots 0 0 0 1 2 2 2
  line L219 (8.3333, -23.0255) -> (8.2618, -23.0547)
  line L220 (8.2618, -23.0547) -> (8.0237, -22.4715)
  spline S155 degree 2 poles (8.0237, -22.4715) (8.144, -22.3824) (8.4307, -22.2186) (8.6536, -22.1276) knots 0 0 0 1 2 2 2
  line L221 (7.2069, -24.6526) -> (8.0706, -24.3835)
  line L222 (8.0706, -24.3835) -> (8.37, -25.3444)
  line L223 (8.37, -25.3444) -> (7.5064, -25.6136)
  line L224 (7.5064, -25.6136) -> (7.2069, -24.6526)
  line L225 (6.6512, -22.8693) -> (7.5149, -22.6001)
  line L226 (7.5149, -22.6001) -> (7.8143, -23.5611)
  line L227 (7.8143, -23.5611) -> (6.9506, -23.8302)
  line L228 (6.9506, -23.8302) -> (6.6512, -22.8693)
  spline S156 degree 2 poles (1.7716, -24.9449) (1.7358, -24.6662) (1.8823, -24.1835) (2.0609, -23.9987) knots 0 0 0 1 2 2 2
  spline S157 degree 2 poles (2.0609, -23.9987) (2.2395, -23.8139) (2.7595, -23.5728) (3.1484, -23.5228) knots 0 0 0 1 2 2 2
  spline S158 degree 2 poles (3.1484, -23.5228) (3.5894, -23.4661) (4.2391, -23.5321) (4.45, -23.5984) knots 0 0 0 1 2 2 2
  line L229 (4.45, -23.5984) -> (4.5554, -24.4191)
  line L230 (4.5554, -24.4191) -> (4.4636, -24.4309)
  spline S159 degree 2 poles (4.4636, -24.4309) (4.2384, -24.3259) (3.6528, -24.202) (3.4201, -24.2319) knots 0 0 0 1 2 2 2
  spline S160 degree 2 poles (3.4201, -24.2319) (3.2823, -24.2496) (2.967, -24.3399) (2.867, -24.4337) knots 0 0 0 1 2 2 2
  spline S161 degree 2 poles (2.867, -24.4337) (2.7895, -24.509) (2.7094, -24.7092) (2.731, -24.8776) knots 0 0 0 1 2 2 2
  spline S162 degree 2 poles (2.731, -24.8776) (2.7527, -25.046) (2.9229, -25.2078) (3.0509, -25.235) knots 0 0 0 1 2 2 2
  spline S163 degree 2 poles (3.0509, -25.235) (3.1789, -25.2621) (3.52, -25.2276) (3.6517, -25.2107) knots 0 0 0 1 2 2 2
  line L231 (3.6517, -25.2107) -> (3.814, -25.1898)
  line L232 (3.814, -25.1898) -> (3.8994, -25.8544)
  line L233 (3.8994, -25.8544) -> (3.7493, -25.8736)
  spline S164 degree 2 poles (3.7493, -25.8736) (3.5778, -25.8957) (3.2908, -25.9637) (3.1957, -26.0226) knots 0 0 0 1 2 2 2
  spline S165 degree 2 poles (3.1957, -26.0226) (3.1009, -26.0846) (3.0096, -26.2706) (3.0285, -26.4176) knots 0 0 0 1 2 2 2
  spline S166 degree 2 poles (3.0285, -26.4176) (3.0435, -26.534) (3.1692, -26.6642) (3.2508, -26.6941) knots 0 0 0 1 2 2 2
  spline S167 degree 2 poles (3.2508, -26.6941) (3.3486, -26.7283) (3.5975, -26.7274) (3.6833, -26.7164) knots 0 0 0 1 2 2 2
  spline S168 degree 2 poles (3.6833, -26.7164) (3.8211, -26.6987) (4.1037, -26.597) (4.2318, -26.5276) knots 0 0 0 1 2 2 2
  spline S169 degree 2 poles (4.2318, -26.5276) (4.3339, -26.474) (4.5501, -26.3155) (4.6009, -26.2747) knots 0 0 0 1 2 2 2
  line L234 (4.6009, -26.2747) -> (4.6805, -26.2645)
  line L235 (4.6805, -26.2645) -> (4.7844, -27.073)
  spline S170 degree 2 poles (4.7844, -27.073) (4.599, -27.1808) (3.9576, -27.422) (3.6115, -27.4665) knots 0 0 0 1 2 2 2
  spline S171 degree 2 poles (3.6115, -27.4665) (3.2747, -27.5098) (2.7636, -27.4571) (2.5745, -27.3662) knots 0 0 0 1 2 2 2
  spline S172 degree 2 poles (2.5745, -27.3662) (2.3663, -27.2716) (2.1261, -26.9289) (2.0966, -26.6992) knots 0 0 0 1 2 2 2
  spline S173 degree 2 poles (2.0966, -26.6992) (2.0549, -26.3746) (2.3663, -25.8428) (2.6635, -25.733) knots 0 0 0 1 2 2 2
  line L236 (2.6635, -25.733) -> (2.6588, -25.6962)
  spline S174 degree 2 poles (2.6588, -25.6962) (2.5217, -25.6952) (2.2519, -25.6302) (2.1152, -25.5357) knots 0 0 0 1 2 2 2
  spline S175 degree 2 poles (2.1152, -25.5357) (1.9893, -25.4523) (1.7991, -25.1592) (1.7716, -24.9449) knots 0 0 0 1 2 2 2
  line L237 (0.1082, -23.8165) -> (1.0126, -23.7953)
  line L238 (1.0126, -23.7953) -> (1.0363, -24.8015)
  line L239 (1.0363, -24.8015) -> (0.1319, -24.8228)
  line L240 (0.1319, -24.8228) -> (0.1082, -23.8165)
  spline S176 degree 2 poles (-3.5401, -25.515) (-3.5002, -25.0226) (-3.2834, -24.2967) (-3.0878, -24.0616) knots 0 0 0 1 2 2 2
  spline S177 degree 2 poles (-3.0878, -24.0616) (-2.8955, -23.8294) (-2.318, -23.6222) (-1.918, -23.6546) knots 0 0 0 1 2 2 2
  spline S178 degree 2 poles (-1.918, -23.6546) (-1.5148, -23.6873) (-0.9813, -23.9845) (-0.8264, -24.251) knots 0 0 0 1 2 2 2
  spline S179 degree 2 poles (-0.8264, -24.251) (-0.6711, -24.5145) (-0.5735, -25.2597) (-0.6134, -25.7521) knots 0 0 0 1 2 2 2
  spline S180 degree 2 poles (-0.6134, -25.7521) (-0.6543, -26.2568) (-0.8691, -26.958) (-1.0685, -27.2021) knots 0 0 0 1 2 2 2
  spline S181 degree 2 poles (-1.0685, -27.2021) (-1.2675, -27.4399) (-1.8506, -27.6405) (-2.2383, -27.6091) knots 0 0 0 1 2 2 2
  spline S182 degree 2 poles (-2.2383, -27.6091) (-2.6476, -27.5759) (-3.1745, -27.2731) (-3.3292, -27.0034) knots 0 0 0 1 2 2 2
  spline S183 degree 2 poles (-3.3292, -27.0034) (-3.4813, -26.7402) (-3.5787, -25.992) (-3.5401, -25.515) knots 0 0 0 1 2 2 2
  spline S184 degree 2 poles (-2.583, -25.5925) (-2.6401, -26.2972) (-2.4554, -26.8853) (-2.1815, -26.9074) knots 0 0 0 1 2 2 2
  spline S185 degree 2 poles (-2.1815, -26.9074) (-1.9076, -26.9296) (-1.6276, -26.3793) (-1.5703, -25.6714) knots 0 0 0 1 2 2 2
  spline S186 degree 2 poles (-1.5703, -25.6714) (-1.5139, -24.9759) (-1.7009, -24.3784) (-1.9748, -24.3563) knots 0 0 0 1 2 2 2
  spline S187 degree 2 poles (-1.9748, -24.3563) (-2.2456, -24.3343) (-2.5264, -24.8939) (-2.583, -25.5925) knots 0 0 0 1 2 2 2
  line L241 (-5.5248, -27.2379) -> (-5.0676, -25.794)
  line L242 (-5.0676, -25.794) -> (-4.5536, -25.9006)
  line L243 (-4.5536, -25.9006) -> (-4.7086, -27.4073)
  line L244 (-4.7086, -27.4073) -> (-5.5248, -27.2379)
  line L245 (-6.5799, -27.019) -> (-6.1226, -25.5751)
  line L246 (-6.1226, -25.5751) -> (-5.6087, -25.6817)
  line L247 (-5.6087, -25.6817) -> (-5.7636, -27.1884)
  line L248 (-5.7636, -27.1884) -> (-6.5799, -27.019)
  line L249 (-12.3479, -24.7721) -> (-9.6629, -21.7686)
  line L250 (-9.6629, -21.7686) -> (-8.7438, -22.1556)
  line L251 (-8.7438, -22.1556) -> (-9.0157, -26.1751)
  line L252 (-9.0157, -26.1751) -> (-9.9291, -25.7905)
  line L253 (-9.9291, -25.7905) -> (-9.6918, -23.0864)
  line L254 (-9.6918, -23.0864) -> (-11.4572, -25.1471)
  line L255 (-11.4572, -25.1471) -> (-12.3479, -24.7721)
  spline S188 degree 2 poles (-15.909, -20.2595) (-15.6266, -19.8542) (-15.0737, -19.3363) (-14.7863, -19.2318) knots 0 0 0 1 2 2 2
  spline S189 degree 2 poles (-14.7863, -19.2318) (-14.5032, -19.128) (-13.9, -19.2398) (-13.5707, -19.4693) knots 0 0 0 1 2 2 2
  spline S190 degree 2 poles (-13.5707, -19.4693) (-13.2389, -19.7006) (-12.9277, -20.2261) (-12.9281, -20.5344) knots 0 0 0 1 2 2 2
  spline S191 degree 2 poles (-12.9281, -20.5344) (-12.9267, -20.8402) (-13.2176, -21.5331) (-13.5001, -21.9384) knots 0 0 0 1 2 2 2
  spline S192 degree 2 poles (-13.5001, -21.9384) (-13.7896, -22.3538) (-14.3284, -22.8514) (-14.6236, -22.9618) knots 0 0 0 1 2 2 2
  spline S193 degree 2 poles (-14.6236, -22.9618) (-14.9153, -23.0671) (-15.52, -22.9467) (-15.8392, -22.7243) knots 0 0 0 1 2 2 2
  spline S194 degree 2 poles (-15.8392, -22.7243) (-16.1761, -22.4895) (-16.4787, -21.9625) (-16.4765, -21.6516) knots 0 0 0 1 2 2 2
  spline S195 degree 2 poles (-16.4765, -21.6516) (-16.4754, -21.3476) (-16.1827, -20.6521) (-15.909, -20.2595) knots 0 0 0 1 2 2 2
  spline S196 degree 2 poles (-15.1213, -20.8085) (-15.5255, -21.3886) (-15.6621, -21.9896) (-15.4367, -22.1467) knots 0 0 0 1 2 2 2
  spline S197 degree 2 poles (-15.4367, -22.1467) (-15.2113, -22.3039) (-14.6921, -21.9694) (-14.2861, -21.3868) knots 0 0 0 1 2 2 2
  spline S198 degree 2 poles (-14.2861, -21.3868) (-13.8871, -20.8143) (-13.7478, -20.204) (-13.9732, -20.0469) knots 0 0 0 1 2 2 2
  spline S199 degree 2 poles (-13.9732, -20.0469) (-14.1961, -19.8915) (-14.7205, -20.2335) (-15.1213, -20.8085) knots 0 0 0 1 2 2 2
  line L256 (-17.1945, -16.5288) -> (-15.3509, -18.2415)
  line L257 (-15.3509, -18.2415) -> (-15.8027, -18.7278)
  line L258 (-15.8027, -18.7278) -> (-16.3908, -18.1814)
  line L259 (-16.3908, -18.1814) -> (-17.7631, -19.6586)
  line L260 (-17.7631, -19.6586) -> (-17.1749, -20.2049)
  line L261 (-17.1749, -20.2049) -> (-17.5973, -20.6596)
  spline S200 degree 2 poles (-17.5973, -20.6596) (-17.7262, -20.5398) (-18.0134, -20.3363) (-18.1239, -20.301) knots 0 0 0 1 2 2 2
  spline S201 degree 2 poles (-18.1239, -20.301) (-18.2542, -20.2643) (-18.4945, -20.3234) (-18.6086, -20.4281) knots 0 0 0 1 2 2 2
  line L262 (-18.6086, -20.4281) -> (-19.2193, -19.8607)
  line L263 (-19.2193, -19.8607) -> (-17.0717, -17.5489)
  line L264 (-17.0717, -17.5489) -> (-17.6463, -17.0152)
  line L265 (-17.6463, -17.0152) -> (-17.1945, -16.5288)
  dimension "d145" = 47.625
  constraints: 1 centre point, 1 coincident, 1 other
  measures "d145" diameter of A0
extrude "Text" cut sketch "Sketch26" against normal blind 1.905
split "Split1" plane through (0, 25.4, 0) removes the side toward (0, 1, 0)
equation "\"d103\" = hexDiameter"
equation "\"d110\" = centerLineForSpool"
equation "\"d111\" = centerLineForSpool"
equation "\"d112\" = holeForString"
equation "\"d121\" = centerLineForSpool"
equation "\"d122\" = holeForString"
equation "\"d125\" = knotHoleDiameter"
equation "\"d127\" = holeForString"
equation "\"d128\" = centerLineForSpool"
equation "\"d129\" = knotHoleDiameter"
equation "\"d130\" = knotHoleDepth"
equation "\"d86\" = spoolOverallHeight"
equation "\"d89\" = 0.5 * spoolOverallHeight"
equation "\"centerLineForSpool\" = 0.25 * spoolOverallHeight"
equation "\"holeForString\" = stringDiameter + clearanceForString"
equation "\"stringDiameter\" = 3.048"
equation "\"clearanceForString\" = 2.032"
equation "\"hexShaftDiameter\" = 12.7"
equation "\"clearanceForHexShaft\" = 0.508"
equation "\"hexDiameter\" = hexShaftDiameter + clearanceForHexShaft"
equation "\"spoolInteriorDiameter\" = 38.1"
equation "\"spoolInteriroRadius\" = 0.5 * spoolInteriorDiameter"
equation "\"spoolExteriorDiameter\" = 63.5"
equation "\"spoolExteriorRadius\" = 0.5 * spoolExteriorDiameter"
equation "\"hexHoleChamfer\" = 1.5875"
equation "\"stringHoleCenterFromHexShaft\" = 0.5 * hexDiameter + 0.5 * holeForString"
equation "\"textCircleDiameter\" = 0.75 * spoolExteriorDiameter"
equation "\"textHeight\" = 4.572"
equation "\"textDepth\" = 1.27"
equation "\"spoolOverallHeight\" = 50.8"
equation "\"d114\" = -spoolInteriroRadius"
equation "\"knotHoleDiameter\" = 9.525"
equation "\"d126\" = spoolInteriroRadius"
equation "\"metalWasherID\" = 26.67"
equation "\"metalWasherThickness\" = 0"
equation "\"spacerOD\" = 24.13"
equation "\"spacerThickness\" = 2.54"
equation "\"knotHoleDepth\" = 11.1125"
body "Solid3"
